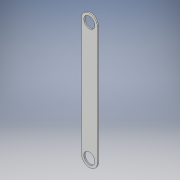
# Autodesk Inventor part: upper-arm-panel
Saved by Autodesk Inventor 2019 (Build 230136000, 136)
## iProperties
Created: 2018-10-19
Part Number: upper-arm-panel
Material: Generic
Document SubType Name: Modeling
Designer: s-2508366
Density: 1 g/cm^3
Appearance: Default
Author: s-2508366
Autodesk Inventor part; units mm, degrees
ref_plane "YZ Plane" through (0, 0, 0) normal (1, 0, 0) x (0, 1, 0)
ref_plane "XZ Plane" through (0, 0, 0) normal (0, 1, 0) x (-1, 0, 0)
ref_plane "XY Plane" through (0, 0, 0) normal (0, 0, 1) x (1, 0, 0)
sketch "Sketch1" plane through (0, 0, 0) normal (0, 0, 1) x (1, 0, 0)
  arc A0 (-20.6375, 0) -> (20.6375, 0) centre (0, 0) ccw
  line L0 (-20.6375, 0) -> (-20.6375, 304.8)
  line L1 (20.6375, 0) -> (20.6375, 304.8)
  arc A1 (20.6375, 304.8) -> (-20.6375, 304.8) centre (0, 304.8) ccw
  circle A2 centre (0, 304.8) radius 14.2875
  circle A3 centre (0, 0) radius 14.2875
  arc A4 (-20.6375, 304.8) -> (20.6375, 304.8) centre (0, 304.8) ccw construction
  arc A5 (20.6375, 0) -> (-20.6375, 0) centre (0, 0) ccw construction
  dimension "d0" = 304.8
  dimension "d2" = 28.575
  dimension "d3" = 6.35
  constraints: 8 point on circle, 6 centre point, 4 end point, 3 coincident, 3 tangent, 2 vertical, 1 equal radius, 1 horizontal alignment
  measures "d0" distance of L1.start L1.end
  measures "d2" diameter of A3
  measures "d3" radial gap between concentric circles of A0 A3
extrude "Extrusion1" add sketch "Sketch1" along normal blind 3.175
body "Solid1"
